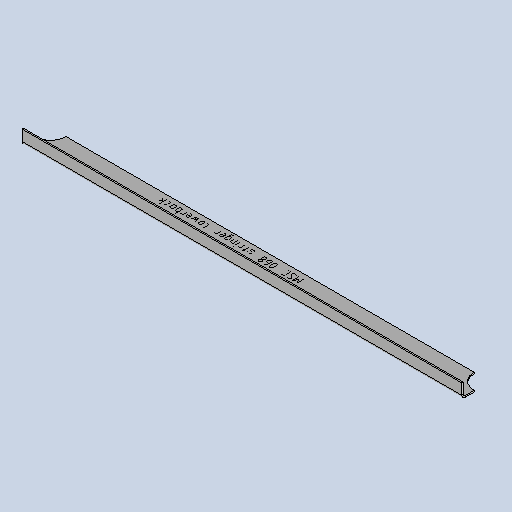
# Autodesk Inventor part: MSC 408 stringer lowerback
Saved by Autodesk Inventor 2025 (Build 290162010, 162A)
## iProperties
Created: 2024-04-28
Part Number: MSC 408 stringer lowerback
Material: Stainless Steel
Document SubType Name: Sheet Metal
Designer: admin
Stock Number: МОО 408 стрингер поясница
Density: 8 g/cm^3
Flat Pattern Width: 62.5 cm
Flat Pattern Length: 5.6202 cm
Flat Pattern Area: 351.262 cm^2
Sheet Metal Rule: AISI304 2mm Die16
Sheet Metal Width: 625,000 mm
Sheet Metal Length: 56,202 mm
Sheet Metal Area: 35126,244 mm^2
Appearance: Default
Author: admin
Autodesk Inventor part; units mm, degrees
ref_plane "YZ Plane" through (0, 0, 0) normal (1, 0, 0) x (0, 1, 0)
ref_plane "XZ Plane" through (0, 0, 0) normal (0, 1, 0) x (-1, 0, 0)
ref_plane "XY Plane" through (0, 0, 0) normal (0, 0, 1) x (1, 0, 0)
sketch "Sketch1" plane through (0, 0, 0) normal (0, 0, 1) x (1, 0, 0)
  line L0 (-625, 40) -> (0, 40)
  line L1 (0, 40) -> (0, 0)
  line L2 (0, 0) -> (-625, 0)
  line L3 (-625, 0) -> (-625, 40)
  point P0 (-312.5, 0)
  dimension "d1" = 40
  dimension "d45" = 625
  measures "d1" distance of L0.end L1.end
  measures "d45" distance of L1.end L2.end
extrude "Plate1" add sketch "Sketch1" along normal blind 2
sketch "Sketch2" plane through (0, 2, 0) normal (0, -1, 0) x (1, 0, 0)
  line L0 (-625, 0) -> (0, 0)
  line L1 (0, 0) -> (0, 20)
  line L2 (0, 20) -> (-625, 20)
  line L3 (-625, 20) -> (-625, 0)
  constraints: 6 end point, 1 horizontal, 1 perpendicular, 1 vertical
edge flange "Flange1" height 20 angle 90 thickness 2 bend radius 2.75 thickness toward (0, -1, 0) relief round relief width 2 relief depth 1 edges at (-312.5, 0, 2) wall of the first edge with corners at (-625, 2, 0) (0, 2, 0) (0, 2, 20) (-625, 2, 20)
bend "Bend1"
corner "Corner1"
sketch "Sketch6" plane through (0, 0, 0) normal (0, 0, -1) x (-1, 0, 0)
  line L0 (0, 40) -> (0, 4.75) projected
  circle A0 centre (0, 40) radius 22.5
  line L1 (0, 40) -> (625, 40) projected
  line L2 (-499, 30) -> (-499, 67.6691) projected
  point P0 (0, 0)
  point P1 (22.5, 40)
  point P2 (0, 17.5)
  dimension "d24" = 45
  constraints: 1 centre point, 1 other
  measures "d24" diameter of A0
extrude "Extrusion2" cut sketch "Sketch6" along normal mid plane 30 contours L1 A0 L0 picked at (14.812, 38.3311)
sketch "Sketch9" plane through (0, 0, 2) normal (0, 0, 1) x (1, 0, 0)
  line L0 (-256.9226, 35) -> (-256.9226, 23) construction
  line L1 (-256.9226, 23) -> (-456.9226, 23) construction
  line L2 (-456.9226, 23) -> (-456.9226, 35) construction
  line L3 (-456.9226, 35) -> (-256.9226, 35) construction
  line L4 (-625, 40) -> (0, 40) projected
  point P0 (0, 0)
  dimension "d40" = 200
  dimension "d41" = 12
  dimension "d43" = 5
  constraints: 2 other
  measures "d40" distance of L0.end L1.end
  measures "d41" distance of L1.end L2.end
  measures "d43" distance between parallel lines of L4 L3
mark "Mark2"
sketch "Sketch10" plane through (-625, 40, 2) normal (0, 0, 1) x (1, 0, 0)
  circle A0 centre (0, 0) radius 22.5
  line L0 (171.5218, -6.4882) -> (171.5218, -9.8215) projected
  line L1 (171.5218, -9.8215) -> (171.5218, -16.4882) projected
  line L2 (171.5218, -9.8215) -> (167.0774, -13.1549) projected
  line L3 (194.8552, -13.1549) -> (194.8552, -6.4882) projected
  line L4 (194.8552, -16.4882) -> (194.8552, -13.1549) projected
  line L5 (192.0774, -13.1549) -> (194.8552, -13.1549) projected
  arc A1 (190.4107, -11.4882) -> (192.0774, -13.1549) centre (192.0774, -11.4882) ccw projected
  line L6 (190.4107, -8.1549) -> (190.4107, -11.4882) projected
  arc A2 (192.0774, -6.4882) -> (190.4107, -8.1549) centre (192.0774, -8.1549) ccw projected
  line L7 (194.8552, -6.4882) -> (192.0774, -6.4882) projected
  line L8 (230.4107, -6.4882) -> (230.9663, -6.4882) projected
  arc A3 (232.6329, -8.1549) -> (230.9663, -6.4882) centre (230.9663, -8.1549) ccw projected
  line L9 (232.6329, -8.1549) -> (232.6329, -16.4882) projected
  circle A4 centre (276.244, -16.2104) radius 0.2778 projected
  line L10 (276.244, -6.4882) -> (276.244, -13.1549) projected
  line L11 (288.744, -6.4882) -> (288.744, -13.1549) projected
  line L12 (289.8552, -13.1549) -> (288.744, -13.1549) projected
  line L13 (288.744, -13.1549) -> (288.744, -16.4882) projected
  line L14 (288.744, -13.1549) -> (286.5218, -13.1549) projected
  line L15 (344.2996, -6.4882) -> (346.5218, -6.4882) projected
  arc A5 (348.744, -8.7104) -> (346.5218, -6.4882) centre (346.5218, -8.7104) ccw projected
  line L16 (348.744, -8.7104) -> (348.744, -14.266) projected
  arc A6 (346.5218, -16.4882) -> (348.744, -14.266) centre (346.5218, -14.266) ccw projected
  line L17 (346.5218, -16.4882) -> (344.2996, -16.4882) projected
  line L18 (367.0774, -6.4882) -> (367.0774, -16.4882) projected
  line L19 (367.0774, -16.4882) -> (363.744, -10.9326) projected
  line L20 (363.744, -10.9326) -> (360.4107, -16.4882) projected
  line L21 (360.4107, -16.4882) -> (360.4107, -6.4882) projected
  arc A7 (357.0774, -7.0437) -> (354.2996, -6.4882) centre (355.0103, -10.157) ccw projected
  arc A8 (354.2996, -6.4882) -> (353.1885, -10.9326) centre (354.3983, -8.874) ccw projected
  line L22 (353.1885, -10.9326) -> (355.9663, -12.5993) projected
  arc A9 (356.5218, -15.9326) -> (355.9663, -12.5993) centre (354.8374, -14.5004) ccw projected
  arc A10 (352.0774, -15.9326) -> (356.5218, -15.9326) centre (354.2996, -11.8029) ccw projected
  arc A11 (327.0774, -15.3771) -> (330.4107, -15.3771) centre (328.744, -14.6897) ccw projected
  arc A12 (327.0774, -7.5993) -> (327.0774, -15.3771) centre (340.5209, -11.4882) ccw projected
  arc A13 (330.4107, -7.5993) -> (327.0774, -7.5993) centre (328.744, -8.308) ccw projected
  arc A14 (330.4107, -15.3771) -> (330.4107, -7.5993) centre (316.9672, -11.4882) ccw projected
  arc A15 (319.8552, -16.4882) -> (323.1885, -10.9326) centre (317.4255, -11.2526) ccw projected
  line L23 (323.1885, -10.9326) -> (323.1885, -8.7104) projected
  arc A16 (323.1885, -8.7104) -> (318.744, -8.7104) centre (320.9663, -8.7104) ccw projected
  line L24 (318.744, -8.7104) -> (318.744, -9.8215) projected
  arc A17 (318.744, -9.8215) -> (320.9663, -12.0437) centre (320.9663, -9.8215) ccw projected
  line L25 (320.9663, -12.0437) -> (322.6329, -12.0437) projected
  line L26 (310.9663, -8.7104) -> (310.9663, -9.8215) projected
  arc A18 (315.4107, -8.7104) -> (310.9663, -8.7104) centre (313.1885, -8.7104) ccw projected
  line L27 (315.4107, -9.8215) -> (315.4107, -8.7104) projected
  arc A19 (313.1885, -12.0437) -> (315.4107, -9.8215) centre (313.1885, -9.8215) ccw projected
  line L28 (313.744, -12.0437) -> (313.1885, -12.0437) projected
  arc A20 (315.4107, -13.7104) -> (313.744, -12.0437) centre (313.744, -13.7104) ccw projected
  line L29 (315.4107, -14.8215) -> (315.4107, -13.7104) projected
  arc A21 (313.744, -16.4882) -> (315.4107, -14.8215) centre (313.744, -14.8215) ccw projected
  line L30 (312.6329, -16.4882) -> (313.744, -16.4882) projected
  arc A22 (310.9663, -14.8215) -> (312.6329, -16.4882) centre (312.6329, -14.8215) ccw projected
  line L31 (310.9663, -13.7104) -> (310.9663, -14.8215) projected
  arc A23 (312.6329, -12.0437) -> (310.9663, -13.7104) centre (312.6329, -13.7104) ccw projected
  line L32 (313.1885, -12.0437) -> (312.6329, -12.0437) projected
  arc A24 (310.9663, -9.8215) -> (313.1885, -12.0437) centre (313.1885, -9.8215) ccw projected
  arc A25 (297.6329, -7.5993) -> (295.9663, -6.4882) centre (295.9544, -8.3116) ccw projected
  line L33 (295.9663, -6.4882) -> (294.8552, -6.4882) projected
  arc A26 (294.8552, -6.4882) -> (293.1885, -7.5993) centre (294.8671, -8.3116) ccw projected
  line L34 (293.1885, -7.5993) -> (293.1885, -8.1549) projected
  arc A27 (293.1885, -8.1549) -> (294.2996, -9.266) centre (295.044, -7.4104) ccw projected
  line L35 (294.2996, -9.266) -> (296.5218, -10.3771) projected
  arc A28 (297.6329, -11.4882) -> (296.5218, -10.3771) centre (295.7774, -12.2326) ccw projected
  line L36 (297.6329, -11.4882) -> (297.6329, -12.0437) projected
  arc A29 (295.9663, -13.1549) -> (297.6329, -12.0437) centre (295.9544, -11.3314) ccw projected
  line L37 (295.9663, -13.1549) -> (294.8552, -13.1549) projected
  arc A30 (293.1885, -12.0437) -> (294.8552, -13.1549) centre (294.8671, -11.3314) ccw projected
  line L38 (283.1885, -6.4882) -> (283.1885, -13.1549) projected
  line L39 (283.1885, -13.1549) -> (280.9663, -13.1549) projected
  arc A31 (279.8552, -12.0437) -> (280.9663, -13.1549) centre (280.9663, -12.0437) ccw projected
  line L40 (272.6329, -6.4882) -> (272.6329, -13.1549) projected
  line L41 (272.6329, -13.1549) -> (269.8552, -13.1549) projected
  arc A32 (268.1885, -11.4882) -> (269.8552, -13.1549) centre (269.8552, -11.4882) ccw projected
  line L42 (268.1885, -11.4882) -> (268.1885, -6.4882) projected
  line L43 (263.1885, -13.1549) -> (260.4107, -13.1549) projected
  line L44 (260.4107, -13.1549) -> (260.4107, -6.4882) projected
  line L45 (260.4107, -6.4882) -> (260.4107, -4.8215) projected
  arc A33 (262.0774, -3.1549) -> (260.4107, -4.8215) centre (262.0774, -4.8215) ccw projected
  line L46 (262.0774, -3.1549) -> (264.8552, -3.1549) projected
  line L47 (260.4107, -6.4882) -> (263.1885, -6.4882) projected
  arc A34 (264.8552, -8.1549) -> (263.1885, -6.4882) centre (263.1885, -8.1549) ccw projected
  line L48 (264.8552, -8.1549) -> (264.8552, -11.4882) projected
  arc A35 (263.1885, -13.1549) -> (264.8552, -11.4882) centre (263.1885, -11.4882) ccw projected
  line L49 (257.0774, -10.9326) -> (257.0774, -9.8215) projected
  arc A36 (252.6329, -10.9326) -> (257.0774, -10.9326) centre (254.8552, -10.9326) ccw projected
  line L50 (252.6329, -9.8215) -> (252.6329, -10.9326) projected
  line L51 (257.0774, -9.8215) -> (252.6329, -9.8215) projected
  line L52 (257.0774, -9.8215) -> (257.0774, -8.1549) projected
  arc A37 (257.0774, -8.1549) -> (255.4107, -6.4882) centre (255.4107, -8.1549) ccw projected
  line L53 (255.4107, -6.4882) -> (252.6329, -6.4882) projected
  line L54 (249.2996, -6.4882) -> (249.2996, -13.1549) projected
  line L55 (249.2996, -13.1549) -> (247.0774, -13.1549) projected
  arc A38 (245.9663, -12.0437) -> (247.0774, -13.1549) centre (247.0774, -12.0437) ccw projected
  arc A39 (222.6329, -10.9326) -> (227.0774, -10.9326) centre (224.8552, -10.9326) ccw projected
  line L56 (222.6329, -8.7104) -> (222.6329, -10.9326) projected
  arc A40 (227.0774, -8.7104) -> (222.6329, -8.7104) centre (224.8552, -8.7104) ccw projected
  line L57 (227.0774, -10.9326) -> (227.0774, -8.7104) projected
  line L58 (219.2996, -13.1549) -> (217.6329, -6.4882) projected
  line L59 (217.6329, -6.4882) -> (215.9663, -10.9326) projected
  line L60 (215.9663, -10.9326) -> (214.2996, -6.4882) projected
  line L61 (214.2996, -6.4882) -> (212.6329, -13.1549) projected
  line L62 (209.2996, -10.9326) -> (209.2996, -9.8215) projected
  arc A41 (204.8552, -10.9326) -> (209.2996, -10.9326) centre (207.0774, -10.9326) ccw projected
  line L63 (204.8552, -9.8215) -> (204.8552, -10.9326) projected
  line L64 (209.2996, -9.8215) -> (204.8552, -9.8215) projected
  line L65 (209.2996, -9.8215) -> (209.2996, -8.1549) projected
  arc A42 (209.2996, -8.1549) -> (207.6329, -6.4882) centre (207.6329, -8.1549) ccw projected
  line L66 (207.6329, -6.4882) -> (204.8552, -6.4882) projected
  line L67 (201.5218, -6.4882) -> (201.5218, -13.1549) projected
  line L68 (201.5218, -13.1549) -> (199.2996, -13.1549) projected
  arc A43 (198.1885, -12.0437) -> (199.2996, -13.1549) centre (199.2996, -12.0437) ccw projected
  line L69 (184.8552, -13.1549) -> (182.6329, -13.1549) projected
  line L70 (182.6329, -13.1549) -> (182.6329, -8.1549) projected
  line L71 (182.6329, -8.1549) -> (182.6329, -7.5993) projected
  arc A44 (182.6329, -7.5993) -> (181.5218, -6.4882) centre (181.5218, -7.5993) ccw projected
  arc A45 (184.2996, -6.4882) -> (182.6329, -8.1549) centre (184.2996, -8.1549) ccw projected
  line L72 (184.2996, -6.4882) -> (185.4107, -6.4882) projected
  arc A46 (187.0774, -8.1549) -> (185.4107, -6.4882) centre (185.4107, -8.1549) ccw projected
  line L73 (187.0774, -8.1549) -> (187.0774, -10.9326) projected
  arc A47 (184.8552, -13.1549) -> (187.0774, -10.9326) centre (184.8552, -10.9326) ccw projected
  line L74 (174.8552, -6.4882) -> (176.5218, -6.4882) projected
  arc A48 (178.1885, -8.1549) -> (176.5218, -6.4882) centre (176.5218, -8.1549) ccw projected
  line L75 (178.1885, -8.1549) -> (178.1885, -11.4882) projected
  arc A49 (176.5218, -13.1549) -> (178.1885, -11.4882) centre (176.5218, -11.4882) ccw projected
  line L76 (176.5218, -13.1549) -> (174.8552, -13.1549) projected
  line L77 (169.8552, -10.9326) -> (167.0774, -6.4882) projected
  arc A50 (602.5, 0) -> (625, -22.5) centre (625, 0) ccw projected
  line L78 (0, 0) -> (602.5, 0) projected
  line L79 (0, -35.25) -> (0, 0) projected
  line L80 (0, -35.25) -> (625, -35.25) projected
  line L81 (625, -22.5) -> (625, -35.25) projected
  point P0 (625, -40)
  point P1 (0, -22.5)
  point P2 (22.5, 0)
  dimension "d46" = 45
  constraints: 1 centre point, 1 coincident
  measures "d46" diameter of A0
extrude "Extrusion4" cut sketch "Sketch10" against normal through all contours A0 L79 L78 picked at (14.812, -1.6689)
equation "\"d43\" = d42"
equation "\"d2\" = Thickness"
equation "\"d3\" = BendReliefWidth"
equation "\"d4\" = BendReliefDepth"
equation "\"d5\" = MinimumRemnant"
equation "\"d6\" = TransitionRadius"
equation "\"d9\" = BendRadius"
equation "\"d10\" = CornerReliefSize"
equation "\"d11\" = GapSize"
equation "\"d12\" = JacobiRadiusSize"
equation "\"BendReliefWidth\" = Thickness"
equation "\"BendReliefDepth\" = 0.5 * Thickness"
equation "\"CornerReliefSize\" = 4 * Thickness"
equation "\"MinimumRemnant\" = 2 * Thickness"
equation "\"TransitionRadius\" = BendRadius"
equation "\"JacobiRadiusSize\" = BendRadius"
equation "\"GapSize\" = Thickness"
equation "\"qqqqqq\" = 67.35706"
equation "\"d42\" = 5"
equation "\"Thickness\" = 2"
equation "\"BendRadius\" = 2.75"
body "Solid1"
